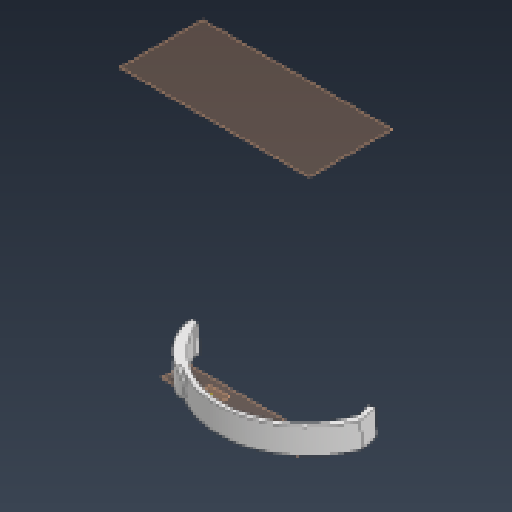
# Autodesk Inventor part: thigh_strap_05
Saved by Autodesk Inventor 2025.2 (Build 292293000, 293)
## iProperties
Created: 2025-03-07
Part Number: thigh_strap_05
Material: Generic
Document SubType Name: Modeling
Designer: email
Density: 1 g/cm^3
Appearance: Default
Author: email
Autodesk Inventor part; units mm, degrees
ref_plane "YZ Plane" through (0, 0, 0) normal (1, 0, 0) x (0, 1, 0)
ref_plane "XY Plane" through (0, 0, 0) normal (0, 0, 1) x (1, 0, 0)
ref_plane "Work Plane1" through (0, -273.05, 0) normal (0, 1, 0) x (-1, 0, 0)
sketch "Sketch1" plane through (0, -273.05, 0) normal (0, 1, 0) x (-1, 0, 0)
  line L0 (28.2313, 0) -> (-81.8149, 0)
  point P0 (0, 0)
  constraints: 2 end point, 1 horizontal
ref_plane "Work Plane2" through (-28.2313, -273.05, 0) normal (0, 0.9994, 0.0349) x (1, 0, 0)
sketch "Sketch2" plane through (-28.2313, -273.05, 0) normal (0, 0.9994, 0.0349) x (1, 0, 0)
  ellipse E0 centre (142.9444, 40.4167) end of major axis (127.2199, 83.6456) minor radius 0.5491 (135.3201, 59.9472) -> (144.2427, 35.2519) ccw projected
  ellipse E1 centre (145.4346, 41.3225) end of major axis (129.7101, 84.5514) minor radius 0.5491 (137.8103, 60.853) -> (146.7329, 36.1577) ccw projected
  line L0 (144.2427, 35.2519) -> (146.7329, 36.1577) projected
  ellipse E2 centre (-15.3961, 31.7454) end of major axis (-31.1205, -11.4836) minor radius 0.5491 (-17.0369, 25.6432) -> (-8.0746, 50.4278) ccw projected
  line L1 (-17.0369, 25.6432) -> (-19.5271, 26.549) projected
  ellipse E3 centre (-17.8862, 32.6512) end of major axis (-33.6107, -10.5778) minor radius 0.5491 (-19.5271, 26.549) -> (-10.5647, 51.3336) ccw projected
  line L2 (-19.5271, 32.4296) -> (-18.2659, 22.0654)
  arc A0 (-18.2659, 22.0654) -> (148.9119, 28.6146) centre (63.7007, 66.7506) ccw
  line L3 (148.9119, 28.6146) -> (145.6991, 46.4313)
  line L4 (145.6991, 46.4313) -> (139.9268, 44.3316)
  line L5 (139.9268, 44.3316) -> (144.0175, 33.0855)
  line L6 (-19.5271, 32.4296) -> (-12.1574, 30.5326)
  line L7 (-12.1574, 30.5326) -> (-12.6035, 26.6966)
  arc A1 (-12.6035, 26.6966) -> (144.0175, 33.0855) centre (64.3823, 62.3675) ccw
  line L8 (24.7417, -18.0874) -> (23.158, -19.0562)
  arc A2 (-20.3945, 31.8123) -> (23.158, -19.0562) centre (36.4902, 36.4371) ccw
  line L9 (-20.3945, 31.8123) -> (-19.5271, 32.4296)
  point P0 (28.2313, 9.5293)
  point P1 (-19.007, 27.8025)
  point P2 (140.8209, 44.6568)
  point P3 (-14.9879, 31.2612)
  point P4 (-17.0369, 25.6432)
  point P5 (-18.7784, 26.2767)
  point P6 (143.311, 45.5626)
  point P7 (-19.5271, 26.549)
  point P8 (-18.9903, 28.0182)
  constraints: 16 end point, 7 point on circle, 3 centre point, 1 perpendicular, 1 point on line, 6 other
extrude "Extrusion1" add sketch "Sketch2" along normal blind 25.4
fillet "Fillet1" radius 12.7 2 edges at (-4.2815, -248.3136, 19.4469) (-4.2815, -273.6981, 18.5605)
body "Solid1"
